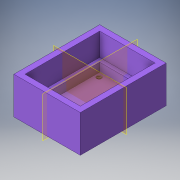
# Autodesk Inventor part: CaseForADXL_345
Saved by Autodesk Inventor 2016 SP1 (Build 200210100, 210)
## iProperties
Created: 2016-02-02
Part Number: CaseForADXL_345
Material: ABS Plastic
Document SubType Name: Modeling
Designer: steele
Density: 1.06 g/cm^3
Appearance: Violet
Author: steele
Autodesk Inventor part; units mm, degrees
ref_plane "XZ Plane" through (0, 0, 0) normal (0, 1, 0) x (-1, 0, 0)
sketch "Sketch3" plane through (0, 0, 0) normal (0, 1, 0) x (-1, 0, 0)
  line L0 (15.24, 19.685) -> (-15.24, 19.685)
  line L1 (-15.24, 19.685) -> (-15.24, -19.685)
  line L2 (-15.24, -19.685) -> (15.24, -19.685)
  line L3 (15.24, -19.685) -> (15.24, 19.685)
  line L4 (15.24, 19.685) -> (-15.24, -19.685) construction
  line L5 (-15.24, 19.685) -> (15.24, -19.685) construction
  line L6 (-12.7, 17.145) -> (-12.7, -17.145)
  line L7 (-12.7, -17.145) -> (12.7, -17.145)
  line L8 (12.7, -17.145) -> (12.7, 17.145)
  line L9 (12.7, 17.145) -> (-12.7, 17.145)
  line L10 (-12.7, 17.145) -> (12.7, -17.145) construction
  line L11 (-12.7, -17.145) -> (12.7, 17.145) construction
  point P0 (0, 0)
  dimension "d11" = 30.48
  dimension "d12" = 39.37
  dimension "d13" = 34.29
  dimension "d14" = 25.4
  constraints: 24 end point, 4 midpoint, 4 parallel, 2 perpendicular, 1 horizontal, 1 vertical
  measures "d11" distance of L0.start L0.end
  measures "d12" distance of L2.end L0.start
  measures "d13" distance of L6.start L6.end
  measures "d14" distance of L8.end L6.start
extrude "Extrusion4" add sketch "Sketch3" along normal blind 16.9926
sketch "Sketch4" plane through (0, 0, 0) normal (0, -1, 0) x (1, 0, 0)
  line L0 (12.7, 17.145) -> (-12.7, 17.145) projected
  line L1 (-12.7, -17.145) -> (12.7, -17.145) projected
  line L2 (12.7, 17.145) -> (-12.7, 17.145)
  line L3 (-12.7, 17.145) -> (-12.7, -17.145)
  line L4 (-12.7, -17.145) -> (12.7, -17.145)
  line L5 (12.7, -17.145) -> (12.7, 17.145)
  point P0 (0, 0)
  constraints: 8 end point, 2 parallel, 1 horizontal, 1 perpendicular
extrude "Extrusion5" add sketch "Sketch4" against normal blind 2.54
sketch "Sketch5" plane through (0, 2.54, 0) normal (0, 1, 0) x (1, 0, 0)
  line L0 (10.795, -15.24) -> (10.795, 15.24)
  line L1 (10.795, 15.24) -> (-10.795, 15.24)
  line L2 (-10.795, 15.24) -> (-10.795, -15.24)
  line L3 (-10.795, -15.24) -> (10.795, -15.24)
  line L4 (10.795, -15.24) -> (-10.795, 15.24) construction
  line L5 (10.795, 15.24) -> (-10.795, -15.24) construction
  line L6 (12.7, -17.145) -> (-12.7, -17.145) projected
  line L7 (12.7, 17.145) -> (12.7, -17.145) projected
  line L8 (-12.7, 17.145) -> (12.7, 17.145) projected
  line L9 (12.7, -17.145) -> (-12.7, -17.145)
  line L10 (-12.7, -17.145) -> (-12.7, 17.145)
  line L11 (-12.7, 17.145) -> (12.7, 17.145)
  line L12 (12.7, 17.145) -> (12.7, -17.145)
  point P0 (0, 0)
  dimension "d21" = 1.905
  dimension "d22" = 1.905
  constraints: 20 end point, 4 parallel, 2 midpoint, 2 perpendicular, 1 horizontal, 1 vertical
  measures "d21" distance between parallel lines of L6 L3
  measures "d22" distance between parallel lines of L7 L0
extrude "Extrusion6" add sketch "Sketch5" along normal blind 3.9878
sketch "Sketch6" plane through (0, 0, 0) normal (0, -1, 0) x (1, 0, 0)
  line L0 (15.24, 19.685) -> (15.24, -19.685) construction
  line L1 (15.24, -13.081) -> (-15.24, -13.081) construction
  line L2 (-15.24, -19.685) -> (-15.24, 19.685) construction
  line L3 (15.24, -19.685) -> (-15.24, -19.685) construction
  point P0 (0, 0)
  point P1 (8.89, -13.081)
  point P2 (-8.89, -13.081)
  dimension "d25" = 6.604
  dimension "d26" = 6.35
  dimension "d27" = 6.35
  constraints: 4 point on line, 2 end point, 1 horizontal
  measures "d25" distance between parallel lines of L1 L3
  measures "d26" distance from line of point (8.89, -13.081) L0
  measures "d27" distance from line of L2 point (-8.89, -13.081)
hole "Hole1" at (8.89, 0, -13.081) at (-8.89, 0, -13.081) direction (0, 1, 0) diameter 2.159 end through all
equation "\"d11\" = caseWidth"
equation "\"d12\" = caseLength"
equation "\"d13\" = internalCaseLength"
equation "\"d14\" = internalCaseWidth"
equation "\"d17\" = caseHeight"
equation "\"d19\" = caseBaseThickness"
equation "\"d21\" = supportWidth"
equation "\"d22\" = supportWidth"
equation "\"d23\" = componentHeightAboveBoard"
equation "\"boardWidth\" = 22.86"
equation "\"boardLength\" = 31.75"
equation "\"boardThickness\" = 1.7272"
equation "\"componentHeightAboveBoard\" = 3.9878"
equation "\"headerHeightAboveBard\" = 8.7376"
equation "\"holeDiam\" = 2.3368"
equation "\"centerLineForHoles\" = 2.794"
equation "\"holeDistanceFromEdge\" = 2.54"
equation "\"supportWidth\" = 1.905"
equation "\"caseWallWidth\" = 2.54"
equation "\"internalSpacingForComponent\" = 1.27"
equation "\"caseWidth\" = 2 * caseWallWidth + boardWidth + 2 * internalSpacingForComponent"
equation "\"caseLength\" = 2 * caseWallWidth + boardLength + 2 * internalSpacingForComponent"
equation "\"internalCaseWidth\" = boardWidth + 2 * internalSpacingForComponent"
equation "\"internalCaseLength\" = boardLength + 2 * internalSpacingForComponent"
equation "\"caseHeight\" = headerHeightAboveBard + boardThickness + componentHeightAboveBoard + caseBaseThickness"
equation "\"caseBaseThickness\" = 2.54"
body "Solid3"
